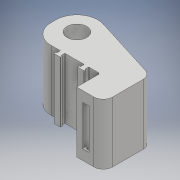
# Autodesk Inventor part: taig_sp2
Saved by Autodesk Inventor 2018 (Build 220112000, 112)
## iProperties
Created: 2018-11-11
Part Number: taig_sp2
Material: Generic
Document SubType Name: Modeling
Designer: svaft
Density: 1 g/cm^3
Appearance: Default
Author: svaft
## iProperties of the stored document taig_sp2_3DPrint.ipt
Created: 2018-11-11
Part Number: taig_sp2_3DPrint
Material: Generic
Document SubType Name: Modeling
Designer: svaft
Density: 1 g/cm^3
Appearance: Default
Author: svaft
Autodesk Inventor part; units mm, degrees
ref_plane "YZ Plane" through (0, 0, 0) normal (1, 0, 0) x (0, 1, 0)
ref_plane "XZ Plane" through (0, 0, 0) normal (0, 1, 0) x (-1, 0, 0)
ref_plane "XY Plane" through (0, 0, 0) normal (0, 0, 1) x (1, 0, 0)
sketch "Sketch1" plane through (0, 0, 0) normal (0, 0, 1) x (1, 0, 0)
  line L0 (-89.2357, 1.25) -> (12.7643, 1.25)
  line L1 (12.7643, 1.25) -> (12.7643, 26.25)
  line L2 (-89.2357, 27.5) -> (-89.2357, 1.25)
  arc A0 (-66.7357, 50) -> (-89.2357, 27.5) centre (-66.7357, 27.5) ccw
  arc A1 (-60.0301, 48.9775) -> (-66.7357, 50) centre (-66.7357, 27.5) ccw
  line L3 (12.7643, 26.25) -> (-60.0301, 48.9775)
  point P0 (0, 0)
  dimension "d34" = 45
  dimension "d35" = 22.5
  dimension "d36" = 102
  dimension "d103" = 25
  constraints: 8 end point, 5 point on circle, 2 centre point, 1 coincident, 1 concentric, 1 horizontal, 1 parallel, 1 perpendicular, 1 tangent
  measures "d34" diameter of A0
  measures "d35" distance from line of L2 A0.centre
  measures "d36" distance between parallel lines of L2 L1
  measures "d103" distance of L0.end L1.end
extrude "Extrusion1" add sketch "Sketch1" along normal blind 65
sketch "Sketch2" plane through (0, 0, 0) normal (0, 0, -1) x (-1, 0, 0)
  line L0 (-10.6787, 5.25) -> (87.2357, 5.25)
  line L1 (87.2357, 5.25) -> (87.2357, 27.5)
  line L2 (89.2357, 27.5) -> (89.2357, 1.25) projected
  line L3 (-12.7643, 1.25) -> (-12.7643, 26.25) projected
  line L4 (89.2357, 1.25) -> (-12.7643, 1.25) projected
  line L5 (-12.7643, 26.25) -> (60.0301, 48.9775) projected
  line L6 (-10.6787, 24.8059) -> (78.3968, 52.6167)
  arc A0 (89.2357, 27.5) -> (60.0301, 48.9775) centre (66.7357, 27.5) ccw projected
  arc A1 (87.2357, 27.5) -> (61.75, 47.3845) centre (66.7357, 27.5) ccw
  line L7 (61.75, 47.3845) -> (-10.6787, 24.8059)
  line L8 (66.7357, 48) -> (63.6099, 48)
  line L9 (57.4621, 48) -> (56.8991, 48)
  line L10 (-10.7961, 26.8645) -> (-10.7961, 50.113)
  line L11 (-10.6787, 24.8059) -> (-10.6787, 5.25)
  point P0 (0, 0)
  point P1 (87.2357, 36.7736)
  dimension "d30" = 2
  dimension "d33" = 4
  dimension "d37" = 2
  dimension "d38" = 2
  constraints: 16 end point, 5 parallel, 5 point on circle, 4 perpendicular, 3 point on line, 2 horizontal, 1 centre point, 1 other
  measures "d30" distance between parallel lines of L2 L1
  measures "d37" distance between parallel lines of L5 L6
  measures "d38" radial gap between concentric circles of A0 A1
extrude "Extrusion2" cut sketch "Sketch2" against normal blind 59 contours L11 L7 A1 L1 L0
sketch "Sketch3" plane through (0, 0, 59) normal (0, 0, -1) x (-1, 0, 0)
  circle A0 centre (66.7357, 26.25) radius 20.2
  circle A1 centre (66.7357, 26.25) radius 22.7
  line L0 (89.2357, 1.25) -> (-12.7643, 1.25) projected
  line L1 (89.2357, 27.5) -> (89.2357, 1.25) projected
  point P0 (0, 0)
  point P1 (-12.7643, 1.25)
  dimension "d6" = 40.4
  dimension "d7" = 2.5
  dimension "d8" = 25
  dimension "d9" = 22.5
  dimension "d27" = 45.4
  constraints: 2 centre point, 1 other
  measures "d6" diameter of A0
  measures "d7" radial gap between concentric circles of A0 A1
  measures "d9" distance from line of L1 A0.centre
  measures "d27" diameter of A1
extrude "Extrusion3" add sketch "Sketch3" along normal blind 40
sketch "Sketch4" plane through (-66.7357, 26.25, 59) normal (0, 0, -1) x (-1, 0, 0)
  circle A0 centre (0, 1.25) radius 20.5 projected
  circle A1 centre (0, 1.25) radius 10.5
  circle A2 centre (0, 0) radius 20.2 projected
  circle A3 centre (0, 0) radius 20.2 projected
  point P0 (-66.7357, -26.25)
  point P1 (20.5, 0)
  dimension "d12" = 21
  constraints: 2 horizontal alignment, 1 centre point, 1 coincident, 1 other
  measures "d12" diameter of A1
extrude "Extrusion4" cut sketch "Sketch4" against normal blind 55 contours A1
sketch "Sketch5" plane through (0, 0, 59) normal (0, 0, -1) x (-1, 0, 0)
  line L0 (-26.0535, 9.1985) -> (-25.8585, 7.6104)
  line L1 (44.116, 16.2022) -> (43.921, 17.7903)
  line L2 (-26.0535, 9.1985) -> (-24.4535, 9.1985) construction
  line L3 (42.4322, 17.6075) -> (42.3094, 18.6075)
  line L4 (42.3094, 18.6075) -> (45.2358, 18.9668)
  arc A0 (75.3548, 5.25) -> (58.1165, 5.25) centre (66.7357, 26.25) ccw projected
  line L5 (42.6272, 16.0194) -> (42.7499, 15.0194)
  line L6 (42.7499, 15.0194) -> (46.7376, 15.5091)
  arc A1 (75.3548, 5.25) -> (58.1165, 5.25) centre (66.7357, 26.25) ccw projected
  line L7 (-24.5647, 9.3813) -> (-24.6866, 10.3739)
  line L8 (-24.6866, 10.3739) -> (-28.7643, 9.8732)
  line L9 (-24.3697, 7.7933) -> (-24.2478, 6.8007)
  line L10 (-24.2478, 6.8007) -> (-28.7643, 6.2462)
  line L11 (-28.7643, 6.2462) -> (-28.7643, 9.8732)
  line L12 (-28.7643, 5.25) -> (-28.7643, 26.7515) projected
  line L13 (-28.7643, 5.25) -> (-28.7643, 26.7515) projected
  line L14 (43.921, 17.7903) -> (42.4322, 17.6075)
  line L15 (-24.5647, 9.3813) -> (-26.0535, 9.1985)
  line L16 (-25.8585, 7.6104) -> (-24.3697, 7.7933)
  line L17 (42.6272, 16.0194) -> (44.116, 16.2022)
  point P0 (0, 0)
  point P1 (74.8134, 48)
  point P2 (57.4621, 48)
  point P3 (-10.6787, 5.25)
  point P4 (-28.7643, 48)
  point P5 (87.2357, 32.7736)
  point P6 (-28.7643, 26.7515)
  dimension "d15" = 1.6
  dimension "d16" = 83
  dimension "d17" = 70.5
  dimension "d19" = 1
  dimension "d20" = 1
  dimension "d22" = 70.5
  dimension "d23" = 1
  dimension "d24" = 1
  dimension "d28" = 1.5
  dimension "d29" = 1.5
  dimension "d87" = 1.5881
  constraints: 32 end point, 10 perpendicular, 5 parallel, 4 point on line, 2 collinear, 2 vertical, 1 equal length, 1 horizontal, 6 other
  measures "d15" distance of L0.start L0.end
  measures "d16" angle of L0 L2
  measures "d17" distance of L1.start L0.end
  measures "d19" distance of L7.start L7.end
  measures "d20" distance of L9.start L9.end
  measures "d22" distance between parallel lines of L1 L0
  measures "d23" vertical distance of L3.start L3.end
  measures "d24" vertical distance of L5.start L5.end
  measures "d28" distance between parallel lines of L0 L7
  measures "d29" distance between parallel lines of L3 L1
  measures "d87" vertical distance of L1.start L1.end
extrude "Extrusion5" [suppressed]
sketch "Sketch8" plane through (0, 0, 65) normal (0, 0, 1) x (1, 0, 0)
  line L0 (-58.3667, -1.056) -> (-58.3667, 2.5) projected
  line L1 (-53.1851, 2.5) -> (-53.1851, -1.056) projected
  line L2 (-89.2357, 1.25) -> (12.7643, 1.25) projected
  line L3 (-53.3851, 2.5) -> (-53.3851, -2.6)
  line L4 (-58.1667, -2.6) -> (-58.1667, 2.5)
  line L5 (-27.8851, -2.6) -> (-27.8851, 1.25)
  line L6 (-32.6667, 1.25) -> (-32.6667, -2.6)
  line L7 (-53.3851, 2.5) -> (-58.1667, 2.5)
  line L8 (-15.6851, 1.25) -> (12.7643, 1.25)
  line L9 (12.7643, 1.25) -> (12.7643, -23.75)
  line L10 (12.7643, -23.75) -> (-15.6851, -23.75)
  line L11 (-15.6851, -23.75) -> (-15.6851, 1.25)
  line L12 (12.7643, 1.25) -> (12.7643, 26.25) projected
  line L13 (-89.2357, 27.5) -> (-89.2357, 1.25) projected
  line L14 (-27.8851, -2.6) -> (-26.6851, -2.6)
  line L15 (-26.6851, -2.6) -> (-26.6851, -4.7)
  line L16 (-32.6667, -2.6) -> (-33.8667, -2.6)
  line L17 (-33.8667, -2.6) -> (-33.8667, -4.7)
  line L18 (-33.8667, -4.7) -> (-26.6851, -4.7)
  line L19 (-53.3851, -2.6) -> (-52.1851, -2.6)
  line L20 (-52.1851, -2.6) -> (-52.1851, -4.7)
  line L21 (-58.1667, -2.6) -> (-59.3667, -2.6)
  line L22 (-59.3667, -2.6) -> (-59.3667, -4.7)
  line L23 (-59.3667, -4.7) -> (-52.1851, -4.7)
  line L24 (-55.7759, 1.25) -> (-55.7759, -3.6)
  line L25 (-30.2759, 1.25) -> (-30.2759, -3.6)
  point P0 (0, 0)
  point P1 (-58.3667, 1.2424)
  point P2 (-53.1851, 1.2424)
  point P3 (30.7643, 18.4478)
  point P4 (12.7643, 26.25)
  dimension "d72" = 5.1816
  dimension "d73" = 0.2
  dimension "d74" = 0.2
  dimension "d90" = 25
  dimension "d104" = 102
  dimension "d127" = 1.2
  dimension "d128" = 2.1
  dimension "d129" = 1.2
  dimension "d130" = 1.2
  dimension "d131" = 2.1
  dimension "d132" = 1.2
  dimension "d135" = 3.85
  dimension "d136" = 4.7816
  dimension "d137" = 4.7816
  dimension "d139" = 4.7816
  dimension "d140" = 4.7816
  dimension "d141" = 25.5
  constraints: 42 end point, 7 perpendicular, 5 horizontal, 3 collinear, 3 parallel, 2 point on line, 2 vertical, 8 other
  measures "d72" distance between parallel lines of L1 L0
  measures "d73" distance between parallel lines of L1 L3
  measures "d74" distance between parallel lines of L0 L4
  measures "d90" distance of L8.end L9.end
  measures "d104" distance between parallel lines of L9 L13
  measures "d127" distance of L5.start L14.end
  measures "d128" distance of L14.end L15.end
  measures "d129" distance of L6.end L16.end
  measures "d130" distance of L3.end L19.end
  measures "d131" distance of L19.end L20.end
  measures "d132" distance of L4.start L21.end
  measures "d136" distance between parallel lines of L6 L5
  measures "d137" distance between parallel lines of L4 L3
  measures "d139" diameter of L3 L24
  measures "d140" diameter of L6 L25
  measures "d141" distance between parallel lines of L25 L24
extrude "T_fixture" add sketch "Sketch8" against normal blind 65
fillet "Fillet2" radius 0.4 16 edges at (-27.8851, -2.6, 32.5) (-32.6667, -2.6, 32.5) (-53.3851, -2.6, 32.5) (-58.1667, -2.6, 32.5) (-26.6851, -4.7, 32.5) (-33.8667, -4.7, 32.5) (-52.1851, -4.7, 32.5) (-59.3667, -4.7, 32.5) (-52.1851, -2.6, 32.5) (-59.3667, -2.6, 32.5) (-33.8667, -2.6, 32.5) (-26.6851, -2.6, 32.5) (-27.8851, 1.25, 32.5) (-32.6667, 1.25, 32.5) (-53.3851, 1.25, 32.5) (-58.1667, 1.25, 32.5)
sketch "Sketch9" plane through (0, 0, 19) normal (0, 0, -1) x (-1, 0, 0)
  arc A0 (53.8067, 44.9083) -> (87.2357, 16.5012) centre (66.7357, 26.25) ccw projected
  line L0 (50.2619, 38.7834) -> (47.8094, 38.7834)
  arc A1 (53.8067, 44.9083) -> (87.2357, 16.5012) centre (66.7357, 26.25) ccw projected
  line L1 (46.9333, 32.2792) -> (44.851, 32.2792)
  line L2 (46.9333, 32.2792) -> (50.2619, 38.7834)
  line L3 (47.8094, 38.7834) -> (45.6161, 38.7834)
  line L4 (45.6161, 38.7834) -> (43.2419, 32.3366)
  line L5 (43.2419, 32.3366) -> (45.8921, 32.2792)
  point P0 (0, 0)
  point P1 (45.4148, 20.3118)
  constraints: 12 end point, 2 horizontal, 1 midpoint, 1 parallel, 4 other
extrude "Extrusion7" [suppressed]
sketch "Sketch10" plane through (-60.0301, 48.9775, 65) normal (0.2980276, 0.9545572, 0) x (0.9545572, -0.2980276, 0)
  line L0 (32.75, 21.5) -> (17.25, 21.5)
  line L1 (17.25, 21.5) -> (17.25, 48.5)
  line L2 (17.25, 48.5) -> (32.75, 48.5)
  line L3 (32.75, 48.5) -> (32.75, 21.5)
  line L4 (32.75, 21.5) -> (17.25, 48.5) construction
  line L5 (17.25, 21.5) -> (32.75, 48.5) construction
  line L6 (76.2598, 65) -> (0, 65) projected
  line L7 (0, 65) -> (0, 0) projected
  line L8 (76.2598, 0) -> (0, 0) projected
  line L9 (76.2598, 65) -> (76.2598, 0) projected
  point P0 (71.8988, 65)
  point P1 (25, 35)
  dimension "d53" = 15.5
  dimension "d54" = 27
  dimension "d57" = 25
  dimension "d59" = 30
  constraints: 12 end point, 2 midpoint, 2 parallel, 1 horizontal, 1 perpendicular
  measures "d53" distance of L1.end L2.end
  measures "d54" distance of L0.end L1.end
  measures "d57" distance from line of L7 point (25, 35)
  measures "d59" distance from line of L6 point (25, 35)
extrude "Extrusion8" cut sketch "Sketch10" against normal up to surface (2.0327 mm away) contours L0 L1 L2 L3
sketch "Sketch11" plane through (-53.8067, 44.9083, 19) normal (-0.2976093, -0.9546877, 0) x (0.9546877, -0.2976093, 0)
  line L0 (33.7996, -3) -> (5.7996, -3)
  line L1 (5.7996, -3) -> (5.7996, 25)
  line L2 (5.7996, 25) -> (33.7996, 25)
  line L3 (33.7996, 25) -> (33.7996, -3)
  line L4 (33.7996, -3) -> (5.7996, 25) construction
  line L5 (5.7996, -3) -> (33.7996, 25) construction
  point P0 (64.7337, -19)
  point P1 (19.7996, 11)
  dimension "d60" = 28
  dimension "d61" = 28
  constraints: 12 end point, 2 midpoint, 2 parallel, 1 horizontal, 1 perpendicular
  measures "d60" distance of L1.end L2.end
  measures "d61" distance of L0.end L1.end
extrude "Extrusion9" cut sketch "Sketch11" against normal blind 1.5
sketch "Sketch12" plane through (0, 0, 59) normal (0, 0, -1) x (-1, 0, 0)
  line L0 (-10.6787, 24.8059) -> (53.8067, 44.9083) projected
  line L1 (43.4965, 41.6942) -> (44.687, 37.8755)
  line L2 (44.687, 37.8755) -> (28.9719, 32.9766)
  line L3 (28.9719, 32.9766) -> (27.7815, 36.7953)
  line L4 (48.27, 43.1823) -> (21.5387, 34.8492) projected
  line L5 (48.27, 43.1823) -> (21.5387, 34.8492) projected
  line L6 (48.27, 43.1823) -> (47.8235, 44.6143) projected
  line L7 (47.8235, 44.6143) -> (21.0923, 36.2813) projected
  line L8 (21.5387, 34.8492) -> (21.0923, 36.2813) projected
  point P0 (0, 0)
  point P1 (-21.1964, 26.5871)
  point P2 (53.8067, 44.9083)
  dimension "d65" = 4
  dimension "d142" = 5
  constraints: 6 end point, 1 perpendicular, 4 other
  measures "d65" distance of L1.start L1.end
  measures "d142" distance between parallel lines of L1 L6
extrude "Extrusion10" add sketch "Sketch12" along normal up to surface (15 mm away)
sketch "Sketch13" plane through (-21.0923, 36.2813, 44) normal (0, 0, -1) x (-0.9546877, 0.2976093, 0)
  line L0 (6.5391, -5.5) -> (6.5391, -1.5) projected
  line L1 (23, -5.5) -> (6.5391, -5.5)
  line L2 (6.5391, -5.5) -> (6.5391, -2.7)
  line L3 (6.5391, -2.7) -> (23, -2.7)
  line L4 (23, -2.7) -> (23, -5.5)
  point P0 (-30.9342, -28.36)
  dimension "d70" = 2.8
  constraints: 8 end point, 2 parallel, 1 horizontal, 1 perpendicular, 1 point on line
  measures "d70" distance between parallel lines of L3 L1
extrude "Extrusion11" add sketch "Sketch13" along normal blind 2.5
sketch "Sketch15" plane through (0, 0, 59) normal (0, 0, -1) x (-1, 0, 0)
  line L0 (-24.1935, 9.1379) -> (-25.6823, 8.9551) projected
  line L1 (-24.1935, 9.1379) -> (43.3787, 17.4347)
  line L2 (-15.4556, 11.8228) -> (-2.4556, 13.419)
  line L3 (-2.4556, 13.419) -> (-3.2537, 19.919)
  line L4 (-3.2537, 19.919) -> (-16.2537, 18.3228)
  line L5 (-16.2537, 18.3228) -> (-15.4556, 11.8228)
  line L6 (4.5898, 20.882) -> (17.5898, 22.4782)
  line L7 (17.5898, 22.4782) -> (18.3879, 15.9782)
  line L8 (18.3879, 15.9782) -> (5.3879, 14.382)
  line L9 (5.3879, 14.382) -> (4.5898, 20.882)
  line L10 (-25.6823, 8.9551) -> (-25.8773, 10.5432) projected
  line L11 (-25.8773, 10.5432) -> (-24.3885, 10.726) projected
  point P0 (0, 0)
  dimension "d79" = 10.5
  dimension "d80" = 6.5
  dimension "d81" = 13
  dimension "d82" = 13
  dimension "d83" = 31.5
  constraints: 18 end point, 6 parallel, 3 collinear, 2 perpendicular, 2 point on line
  measures "d79" distance between parallel lines of L5 L10
  measures "d80" vertical distance of L4.end L2.start
  measures "d81" horizontal distance of L3.end L4.end
  measures "d82" horizontal distance of L6.start L6.end
  measures "d83" distance between parallel lines of L10 L9
extrude "Extrusion13" [suppressed]
sketch "Sketch16" plane through (0, 0, 0) normal (0, 0, -1) x (-1, 0, 0)
  line L0 (-12.7643, 1.25) -> (-12.7643, -23.75) projected
  line L1 (15.6851, -23.75) -> (15.6851, 1.25) projected
  line L2 (-12.7643, -23.75) -> (15.6851, -23.75) projected
  line L3 (13.6851, 2.5) -> (13.6851, -21.75)
  line L4 (13.6851, -21.75) -> (-10.7643, -21.75)
  line L5 (-10.7643, -21.75) -> (-10.7643, 2.5)
  line L6 (-10.7643, 2.5) -> (-10.7643, 15.2643)
  line L7 (-10.7643, 15.2643) -> (13.6851, 15.2643)
  line L8 (13.6851, 15.2643) -> (13.6851, 2.5)
  line L9 (89.2357, 27.5) -> (89.2357, 1.25) projected
  point P0 (0, 0)
  dimension "d91" = 2
  constraints: 12 end point, 2 perpendicular, 1 vertical, 2 other
  measures "d91" distance between parallel lines of L2 L4
extrude "Extrusion14" cut sketch "Sketch16" against normal up to surface (59 mm away)
sketch "Sketch17" plane through (0, 0, 59) normal (0, 0, -1) x (-1, 0, 0)
  line L0 (11.0103, -21.75) -> (9.4103, -21.75)
  line L1 (9.4103, 28.75) -> (11.0103, 28.75)
  line L2 (13.6851, -21.75) -> (-10.7643, -21.75) projected
  line L3 (9.4103, -20.25) -> (7.4103, -20.25)
  line L4 (7.4103, -20.25) -> (7.4103, -21.75)
  line L5 (11.0103, -20.25) -> (13.6851, -20.25)
  line L6 (13.6851, -21.75) -> (13.6851, 5.25) projected
  line L7 (13.6851, -21.75) -> (7.4103, -21.75)
  line L8 (-10.7643, -21.75) -> (13.6851, -21.75) projected
  line L9 (-10.6787, 24.8059) -> (61.75, 47.3845) projected
  line L10 (9.4103, 28.75) -> (9.4103, 27.25)
  line L11 (7.4103, 27.25) -> (7.4103, 30.4449)
  line L12 (11.0103, 27.25) -> (13.0103, 27.25)
  line L13 (13.0103, 27.25) -> (13.0103, 32.1906)
  line L14 (7.4103, 27.25) -> (9.4103, 27.25)
  line L15 (9.4103, -21.75) -> (9.4103, -20.25)
  line L16 (9.4103, 27.25) -> (9.4103, 28.75)
  line L17 (11.0103, 28.75) -> (11.0103, 27.25)
  line L18 (11.0103, -20.25) -> (11.0103, -21.75)
  line L19 (0.3103, -21.75) -> (1.8103, -21.75)
  line L20 (1.8103, -21.75) -> (1.8103, -18.75)
  line L21 (1.8103, -18.75) -> (0.3103, -18.75)
  line L22 (0.3103, -18.75) -> (0.3103, -21.75)
  point P0 (0, 0)
  dimension "d94" = 1.6
  dimension "d95" = 50.5
  dimension "d96" = 0
  dimension "d97" = 2
  dimension "d98" = 2
  dimension "d101" = 1.5
  dimension "d102" = 1.5
  dimension "d164" = 1.5
  dimension "d165" = 5.6
  dimension "d166" = 3
  constraints: 38 end point, 9 parallel, 7 point on line, 6 perpendicular, 5 collinear, 3 horizontal
  measures "d94" distance of L1.start L1.end
  measures "d95" distance of L1.start L0.end
  measures "d96" distance between parallel lines of L2 L0
  measures "d97" distance of L3.start L3.end
  measures "d98" distance of L12.start L12.end
  measures "d101" distance of L1.start L10.end
  measures "d102" distance of L5.start L0.start
  measures "d164" distance of L21.end L20.end
  measures "d165" distance between parallel lines of L20 L4
  measures "d166" distance of L21.end L19.start
extrude "PCB holder" add sketch "Sketch17" along normal up to surface (59 mm away) contours L2 L18 L5 L6 | L2 L4 L3 L15 | L2 L22 L21 L20
fillet "Fillet3" radius 10 4 edges at (10.6787, 24.8059, 29.5) (12.7643, 26.25, 32.5) (12.7643, -23.75, 32.5) (10.7643, -21.75, 29.5)
fillet "Fillet4" radius 21 2 edges at (-87.2357, 5.25, 29.5) (-89.2357, 1.25, 32.5)
fillet "Fillet5" radius 2 2 edges at (-13.6851, 5.25, 29.5) (-15.6851, 1.25, 32.5)
sketch "Sketch24" plane through (0, 0, 59) normal (0, 0, -1) x (-1, 0, 0)
  line L0 (9.4103, -21.75) -> (9.4103, -20.25) projected
  line L1 (11.0103, -20.25) -> (11.0103, -21.75) projected
  line L2 (9.4103, -21.75) -> (11.0103, -21.75)
  line L3 (11.0103, -21.75) -> (11.0103, 28.75)
  line L4 (11.0103, 28.75) -> (9.4103, 28.75)
  line L5 (9.4103, 28.75) -> (9.4103, -21.75)
  line L6 (13.6851, -20.25) -> (13.6851, -21.75) projected
  line L7 (7.4103, -20.25) -> (7.4103, -21.75) projected
  line L8 (9.4103, -21.75) -> (9.4103, -23.75) projected
  line L9 (-3.6548, 26.9955) -> (61.75, 47.3845) projected
  line L10 (9.4103, -21.75) -> (7.4246, -21.75)
  line L11 (7.4246, -21.75) -> (7.4246, 30.4494)
  line L12 (7.4246, 30.4494) -> (9.4103, 30.4494)
  line L13 (9.4103, 30.4494) -> (9.4103, -21.75)
  line L14 (11.0103, -21.75) -> (11.0103, -20.25) projected
  line L15 (11.0103, -21.75) -> (13.0103, -21.75)
  line L16 (13.0103, -21.75) -> (13.0103, 30.4494)
  line L17 (13.0103, 30.4494) -> (11.0103, 30.4494)
  line L18 (11.0103, 30.4494) -> (11.0103, -21.75)
  point P0 (0, 0)
  point P1 (9.4103, -20.55)
  point P2 (11.0103, -20.55)
  point P3 (8.4103, -20.55)
  point P4 (8.4103, -21.45)
  dimension "d152" = 1.6
  dimension "d153" = 50.5
  constraints: 24 end point, 6 parallel, 3 horizontal, 3 perpendicular, 2 point on line, 1 other
  measures "d152" distance of L4.end L3.end
  measures "d153" distance of L3.end L2.end
extrude "Extrusion22" add sketch "Sketch24" along normal blind 2 contours L10 L11 L12 L13 L5 L0 | L1 L3 L18 L17 L16 L15
sketch "Sketch18" plane through (0, 0, 59) normal (0, 0, -1) x (-1, 0, 0)
  line L0 (9.5141, 48.5397) -> (9.5141, -25.8566)
  line L1 (9.5141, -11.25) -> (2.7141, -11.25)
  line L2 (2.7141, -11.25) -> (2.7141, 1.75)
  line L3 (2.7141, 1.75) -> (9.5141, 1.75)
  line L4 (9.5141, 1.75) -> (9.5141, -11.25)
  line L5 (11.0103, -21.75) -> (9.4103, -21.75) projected
  line L6 (9.5141, 9.75) -> (2.7141, 9.75)
  line L7 (2.7141, 9.75) -> (2.7141, 22.75)
  line L8 (2.7141, 22.75) -> (9.5141, 22.75)
  line L9 (9.5141, 22.75) -> (9.5141, 9.75)
  point P0 (0, 0)
  point P1 (13.6851, -21.75)
  point P2 (-0.7643, -21.75)
  dimension "d108" = 6.8
  dimension "d109" = 13
  dimension "d110" = 10.5
  dimension "d111" = 31.5
  dimension "d112" = 6.8
  dimension "d113" = 13
  constraints: 18 end point, 4 parallel, 2 horizontal, 2 perpendicular, 2 point on line, 1 vertical
  measures "d108" distance of L2.end L3.end
  measures "d109" distance of L1.end L2.end
  measures "d110" distance between parallel lines of L5 L1
  measures "d111" distance between parallel lines of L5 L6
  measures "d112" distance of L6.start L6.end
  measures "d113" distance of L6.end L7.end
extrude "Extrusion16" [suppressed]
sketch "Sketch21" plane through (-53.8067, 44.9083, 19) normal (-0.2976093, -0.9546877, 0) x (0.9546877, -0.2976093, 0)
  line L0 (33.7996, -3) -> (5.7996, -3) projected
  line L1 (24.8457, -3) -> (16.8457, -3)
  line L2 (16.8457, -3) -> (16.8457, -6)
  line L3 (16.8457, -6) -> (24.8457, -6)
  line L4 (24.8457, -6) -> (24.8457, -3)
  point P0 (64.7337, -19)
  dimension "d143" = 8
  dimension "d144" = 3
  constraints: 8 end point, 2 parallel, 1 horizontal, 1 perpendicular, 1 point on line
  measures "d143" distance of L3.end L2.end
  measures "d144" distance of L2.end L1.end
extrude "Extrusion19" add sketch "Sketch21" along normal blind 4
sketch "Sketch22" plane through (-30.0869, 37.514, 16) normal (0.9546877, -0.2976093, 0) x (0, 0, -1)
  line L0 (0, 0) -> (-0.9226, -4)
  line L1 (0, 0) -> (0, -4) projected
  line L2 (-0.9226, -4) -> (0, -4)
  line L3 (0, -4) -> (0, 0)
  point P0 (16, -26.86)
  constraints: 6 end point, 1 collinear, 1 perpendicular
extrude "Extrusion20" add sketch "Sketch22" against normal up to surface (8 mm away)
fillet "Fillet7" [suppressed]
sketch "Sketch23" plane through (-66.7357, 26.25, 59) normal (0, 0, -1) x (-1, 0, 0)
  circle A0 centre (0, 1.25) radius 10.5 projected
  circle A1 centre (0, 0) radius 20.2 projected
  point P0 (-66.7357, -26.25)
extrude "Extrusion21" add sketch "Sketch23" along normal blind 15
fillet "Fillet8" radius 0.4 6 edges at (-11.0103, 5.0997, 57) (-9.4103, 5.0997, 57) (-9.4103, -20.25, 28.5) (-11.0103, -20.25, 28.5) (-7.4103, -20.25, 29.5) (-13.0103, 5.0997, 57)
sketch "Sketch25" plane through (-13.6851, -21.75, 9) normal (0, 1, 0) x (1, 0, 0)
  point P0 (13.6851, 9)
sketch "Sketch26" plane through (-13.6851, -21.75, 9) normal (0, 1, 0) x (1, 0, 0)
  line L0 (11.2748, -2) -> (4.2748, -2)
  line L1 (4.2748, -2) -> (4.2748, -45)
  line L2 (4.2748, -45) -> (11.2748, -45)
  line L3 (11.2748, -45) -> (11.2748, -2)
  line L4 (4.2748, -50) -> (6.2748, -50) projected
  line L5 (2.6748, 9) -> (4.2748, 9) projected
  line L6 (4.2748, -50) -> (4.2748, 9) projected
  point P0 (13.6851, 9)
  point P1 (14.4494, -50)
  point P2 (0, 9)
  point P3 (14.4494, 9)
  point P4 (4.2748, 0)
  dimension "d157" = 5
  dimension "d161" = 7
  dimension "d162" = 43
  constraints: 8 end point, 2 parallel, 1 collinear, 1 horizontal, 1 perpendicular
  measures "d157" distance between parallel lines of L2 L4
  measures "d161" distance of L0.start L0.end
  measures "d162" distance of L2.end L0.start
extrude "Extrusion23" cut sketch "Sketch26" along normal mid plane 5
fillet "Fillet9" radius 0.5 3 edges at (-9.4103, -21.75, 32.5) (-2.4103, -21.75, 32.5) (-4.9103, -21.75, 54)
sketch "Sketch20" plane through (0, 0, 0) normal (0, 0, -1) x (-1, 0, 0)
  line L0 (21.6594, -1.6798) -> (23.4985, -64.2076)
  line L1 (23.4985, -64.2076) -> (-48.5311, -54.3993)
  line L2 (-48.5311, -54.3993) -> (-21.8648, 57.7829)
  line L3 (-21.8648, 57.7829) -> (108.708, 67.5912)
  line L4 (108.708, 67.5912) -> (102.2365, -30.5903)
  line L5 (102.2365, -30.5903) -> (63.7773, -5.3503)
  line L6 (66.2357, 5.25) -> (15.6851, 5.25) projected
  line L7 (21.6594, -1.6798) -> (21.5047, 3.5829)
  line L8 (21.5047, 3.5829) -> (58.3123, 3.5829)
  line L9 (57.7274, 3.5829) -> (63.7773, 3.5829)
  line L10 (63.7773, 3.5829) -> (63.7773, -5.3503)
  point P0 (0, 0)
  point P1 (56.659, 6.2854)
  point P2 (21.4556, 5.25)
  point P3 (15.6851, 5.25)
  constraints: 20 end point, 2 horizontal, 2 point on line, 1 perpendicular, 2 other
sketch "Sketch14" plane through (0, 0, 0) normal (0, 0, -1) x (-1, 0, 0)
  line L0 (6.7007, 41.0378) -> (14.8231, 28.8542)
  line L1 (14.8231, 28.8542) -> (42.6268, 34.946)
  line L2 (42.6268, 34.946) -> (39.3957, 49.6931)
  line L3 (39.3957, 49.6931) -> (90.7554, 60.9461)
  line L4 (90.7554, 60.9461) -> (109.2215, -23.3351)
  line L5 (109.2215, -23.3351) -> (-40.1595, -14.2572)
  line L6 (-40.1595, -14.2572) -> (-43.9084, 34.946)
  line L7 (-43.9084, 34.946) -> (6.7007, 41.0378)
  point P0 (0, 0)
  constraints: 16 end point, 3 perpendicular
equation "\"d24\" = d23"
equation "\"d29\" = d28"
equation "\"d74\" = d73"
equation "\"d59\" = 0.5 * d58"
equation "\"d82\" = d81"
equation "\"d112\" = d108"
equation "\"d113\" = d109"
equation "\"d58\" = 60"
body "Solid1"
